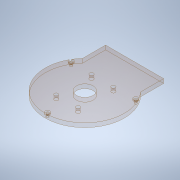
# Autodesk Inventor part: baseSupportCover
Saved by Autodesk Inventor 2022.1 (Build 261234000, 234)
## iProperties
Created: 2020-11-17
Part Number: baseSupportCover
Material: Polycarbonate, Smoke
Document SubType Name: Modeling
Designer: robst
Density: 1.2 g/cm^3
Appearance: Polycarbonate - Smoked
Author: robst
Autodesk Inventor part; units mm, degrees
ref_plane "YZ Plane" through (0, 0, 0) normal (1, 0, 0) x (0, 1, 0)
ref_plane "XZ Plane" through (0, 0, 0) normal (0, 1, 0) x (-1, 0, 0)
ref_plane "XY Plane" through (0, 0, 0) normal (0, 0, 1) x (1, 0, 0)
sketch "Sketch1" plane through (0, 0, 0) normal (0, 1, 0) x (-1, 0, 0)
  arc A0 (38.1, -38.2321) -> (-38.1, -38.2321) centre (0, 0) ccw
  line L0 (0, 0) -> (0, -72.7817) construction
  line L1 (-38.1, -38.2321) -> (-38.1, -69.85)
  line L2 (-38.1, -69.85) -> (0, -69.85)
  line L3 (0, -69.85) -> (38.1, -69.85)
  line L4 (38.1, -69.85) -> (38.1, -38.2321)
  dimension "d0" = 107.95
  dimension "d6" = 69.85
  dimension "d7" = 38.1
  constraints: 10 end point, 2 perpendicular, 2 point on circle, 2 vertical, 1 centre point, 1 coincident, 1 collinear, 1 horizontal, 1 point on line
  measures "d0" diameter of A0
  measures "d6" distance from line of L2 point (0, 0)
  measures "d7" distance between parallel lines of L1 L0
extrude "Extrusion1" add sketch "Sketch1" along normal blind 6.35
sketch "Sketch3" plane through (0, 0, 0) normal (0, -1, 0) x (1, 0, 0)
  arc A0 (38.1, -38.2321) -> (-38.1, -38.2321) centre (0, 0) ccw projected
  line L0 (38.1, -38.2321) -> (38.1, -69.85) projected
  line L1 (38.1, -69.85) -> (-38.1, -69.85) projected
  line L2 (-38.1, -69.85) -> (-38.1, -38.2321) projected
  arc A1 (38.1, -38.2321) -> (-38.1, -38.2321) centre (0, 0) ccw
  line L3 (38.1, -38.2321) -> (38.1, -69.85) projected
  line L4 (38.1, -38.2321) -> (38.1, -69.85)
  line L5 (38.1, -69.85) -> (-38.1, -69.85)
  line L6 (-38.1, -69.85) -> (-38.1, -38.2321) projected
  line L7 (-38.1, -69.85) -> (-38.1, -38.2321)
  arc A2 (44.45, -40.7836) -> (-44.45, -40.7836) centre (0, 0) ccw
  line L8 (44.45, -40.7836) -> (44.45, -76.2)
  line L9 (44.45, -76.2) -> (-44.45, -76.2)
  line L10 (-44.45, -76.2) -> (-44.45, -40.7836)
  dimension "d8" = 6.35
  dimension "d9" = 6.35
  dimension "d10" = 6.35
  dimension "d11" = 6.35
  constraints: 12 end point, 4 point on circle, 2 centre point, 2 coincident, 2 collinear, 2 perpendicular, 2 vertical, 1 concentric
  measures "d8" radial gap between concentric circles of A2 A0
  measures "d9" distance between parallel lines of L8 L0
  measures "d10" distance between parallel lines of L10 L2
  measures "d11" distance between parallel lines of L9 L1
extrude "Extrusion4" add sketch "Sketch3" against normal blind 6.35
sketch "Sketch5" plane through (0, 6.35, 0) normal (0, 1, 0) x (1, 0, 0)
  circle A0 centre (0, 0) radius 12.7
  dimension "d24" = 25.4
  constraints: 1 centre point, 1 coincident
  measures "d24" diameter of A0
extrude "Extrusion7" cut sketch "Sketch5" against normal through all
sketch "Sketch9" plane through (0, 6.35, 0) normal (0, 1, 0) x (1, 0, 0)
  arc A0 (-44.45, 40.7836) -> (44.45, 40.7836) centre (0, 0) ccw construction
  line L0 (-56.0817, 22.225) -> (56.0817, 22.225) construction
  line L1 (-56.0817, -22.225) -> (56.0817, -22.225) construction
  circle A1 centre (0, 0) radius 31.75 construction
  point P0 (-16.7254, -26.9875)
  point P1 (16.7254, -26.9875)
  point P2 (-16.7254, 26.9875)
  point P3 (16.7254, 26.9875)
  dimension "d42" = 22.225
  dimension "d43" = 44.45
  dimension "d44" = 63.5
  dimension "d45" = 4.7625
  dimension "d53" = 53.975
  dimension "d54" = 33.4507
  constraints: 8 point on circle, 4 end point, 2 horizontal, 1 centre point, 1 coincident
  measures "d42" distance from line of L0 point (0, 0)
  measures "d43" distance between parallel lines of L1 L0
  measures "d44" diameter of A1
  measures "d45" distance from line of A1.start L1
  measures "d53" distance of point (-16.725, 26.988) A1.start
  measures "d54" distance of A1.end A1.start
hole "Hole2" at (-16.7254, 6.35, 26.9875) at (16.7254, 6.35, 26.9875) at (-16.7254, 6.35, -26.9875) at (16.7254, 6.35, -26.9875) direction (0, -1, 0) diameter 5.7912 end through all clearance for "Hex Machine Screw" size "#12" standard "Ansi Unified Screw Threads"
sketch "Sketch10" plane through (0, 6.35, 0) normal (0, 1, 0) x (1, 0, 0)
  circle A0 centre (0, 0) radius 57.15 construction
  point P0 (0, -57.15)
  point P1 (49.4934, 28.575)
  point P2 (-49.4934, 28.575)
  dimension "d55" = 114.3
  dimension "d58" = 360
  constraints: 1 coincident, 1 vertical alignment, 6 other
hole "Hole3" at (0, 6.35, 57.15) at (49.4934, 6.35, -28.575) at (-49.4934, 6.35, -28.575) direction (0, -1, 0) diameter 3.81 end through all counterbore diameter 6.858 counterbore depth 2.032 clearance for "Socket Head Cap Screw" size "#6" standard "Ansi Unified Screw Threads"
equation "\"d0\" = exteriorDiameter"
equation "\"d42\" = 0.5 * widthForFork"
equation "\"d43\" = widthForFork"
equation "\"exteriorDiameter\" = 107.95"
equation "\"widthForFork\" = 44.45"
body "Solid1"
